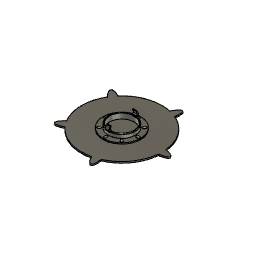
Spool Painting Turntable v16 (Autodesk Fusion 360 design; units mm, degrees)
Autodesk Fusion 360 part; units mm, degrees
sketch "Skizze1" plane through (0, 0, 0) normal (0, 0, 1) x (1, 0, 0)
  circle A0 centre (0, 0) radius 25
  circle A1 centre (0, 0) radius 35
  circle A2 centre (0, 0) radius 75
  dimension "d1" = 50
  dimension "d2" = 10
  dimension "d62" = 150
  constraint coincident A0.centre A1.centre
  measures "d1" diameter of A0
  measures "d62" diameter of A2
ref_plane "Arbeitsebene1" through (0, 0, 38) normal (0, 0, 1) x (1, 0, 0)
extrude "Extrusion1" add sketch "Skizze1" against normal blind 2.5 contours A0 | A1 makes body 1
extrude "Extrusion2" add sketch "Skizze1" along normal blind 2 contours A1 bodies 1
extrude "Extrusion3" add sketch "Skizze1" along normal blind 10 contours A0 bodies 1
ref_plane "Arbeitsebene2" through (0, 0, -0.25) normal (0, 0, 1) x (1, 0, 0)
ref_plane "Arbeitsebene3" through (0, 0, 0.75) normal (0, 0, 1) x (1, 0, 0)
sketch "Skizze3" plane through (0, 0, 0.75) normal (0, 0, 1) x (1, 0, 0)
  line L0 (26.5008, 0) -> (33.4992, 0)
  ellipse E0 centre (30, -0.0006) end of major axis (33.4992, 0.0943) minor radius 2.4634 (26.5008, 0) -> (33.4992, 0) ccw
  spline S0 degree 3 poles (26.2062, 0) (26.2011, -0.4095) (26.3084, -0.8192) (26.5335, -1.1819) (27.1314, -2.1455) (28.4885, -2.7525) (29.8861, -2.7647) (31.1287, -2.7755) (32.3771, -2.3228) (33.1103, -1.5544) (33.5338, -1.1106) (33.7749, -0.5554) (33.795, 0) knots 3.105722 3.105722 3.105722 3.105722 3.531227 3.531227 3.531227 4.661503 4.661503 4.661503 5.666491 5.666491 5.666491 6.246998 6.246998 6.246998 6.246998
  line L1 (26.2062, 0) -> (33.795, 0)
revolve "Drehen5" add sketch "Skizze3" angle 360 about axis through (26.5008, 0, 0.75) along (1, 0, 0) separate body contours L0 E0 L1 makes body 2
revolve "Drehen6" add sketch "Skizze3" angle 360 about axis through (26.2062, 0, 0.75) along (1, 0, 0) separate body makes body 3
pattern_circular "C-Anordnung1" count 8 over 360 about axis through (0, 0, 1.75) along (0, 0, 1) of bodies 3 2 makes body 4 at (22.2285, 20.1064, -1.2055) makes body 5 at (0.3217, 29.9358, 3.1938) makes body 6 at (-21.6185, 20.7163, -1.6309) makes body 7 at (-29.9358, -0.638, 3.1309) makes body 8 at (-19.4839, -22.851, 1.388) makes body 9 at (-0.3217, -29.9358, 3.1938) makes body 10 at (20.1064, -22.2285, -1.2055) makes body 11 at (22.6983, 19.5962, -0.9331) makes body 12 at (2.1935, 29.9035, -0.9331) makes body 13 at (-19.5962, 22.6983, -0.9331) makes body 14 at (-29.9035, -0.7156, -1.9206) makes body 15 at (-19.9571, -22.3374, -1.4435) makes body 16 at (-2.1935, -29.9035, -0.9331) makes body 17 at (19.5962, -22.6983, -0.9331)
combine "Kombinieren3" operation cut target body 1 tool bodies 3 14 17 16 15 12 13 11
fillet "Abrundung1" radius 1.75 1 edges at (-23.3082, -9.0404, 10) on bodies 1
sketch "Skizze5" plane through (0, 0, 10) normal (0, 0, 1) x (-1, 0, 0)
  circle A0 centre (0, 0) radius 23.25
  circle A1 centre (0, 0) radius 23
  dimension "d34" = 46
  constraint coincident A0.centre A1.centre
  measures "d34" diameter of A1
extrude "Extrusion6" cut sketch "Skizze5" against normal up to surface (10.5 mm away) contours A1 bodies 1
fillet "Abrundung4" radius 0.75 1 edges at (21.4435, -8.3172, 10) on bodies 1
ref_plane "Arbeitsebene4" through (0, 0, -1.7) normal (0, 0, -1) x (-1, 0, 0)
sketch "Skizze6" plane through (0, 0, -1.7) normal (0, 0, -1) x (1, 0, 0)
  line L0 (-34, 0.2) -> (-26, 0.2)
  line L1 (-26, 0.2) -> (-26, -0.2)
  line L2 (-26, -0.2) -> (-34, -0.2)
  line L3 (-34, -0.2) -> (-34, 0.2)
  line L4 (-30.2, 3) -> (-29.8, 3)
  line L5 (-29.8, 3) -> (-29.8, -3)
  line L6 (-29.8, -3) -> (-30.2, -3)
  line L7 (-30.2, -3) -> (-30.2, 3)
  constraint horizontal L0
  constraint vertical L1
  constraint horizontal L2
  constraint vertical L3
  constraint horizontal L4
  constraint vertical L5
  constraint horizontal L6
  constraint vertical L7
extrude "Extrusion8" add sketch "Skizze6" against normal blind 0.2 separate body makes body 18
pattern_circular "C-Anordnung3" count 8 over 360 about axis through (0, 0, 1.75) along (0, 0, 1) of bodies 18 makes body 19 at (-19.2333, -19.3276, -1.7) makes body 20 at (0.0667, -32.7333, -1.7) makes body 21 at (19.3276, -19.2333, -1.7) makes body 22 at (31.4667, -0.0667, -1.7) makes body 23 at (19.2333, 19.3276, -1.7) makes body 24 at (-0.0667, 32.7333, -1.7) makes body 25 at (-19.3276, 19.2333, -1.7)
sketch "Skizze7" plane through (0, 0, 0) normal (1, 0, 0) x (0, 1, 0)
  line L0 (25, 8) -> (25, 9.8126)
  line L1 (25.1778, 10.0593) -> (27.8222, 10.9407)
  line L2 (28, 11.1874) -> (28, 11.9386)
  line L3 (27.9726, 12.0549) -> (25.0719, 17.8563)
  line L4 (24.8393, 18) -> (23.4207, 18)
  line L5 (23.1881, 17.6237) -> (25.8659, 12.2681)
  line L6 (25.7156, 11.9052) -> (23.1778, 11.0593)
  line L7 (23, 10.8126) -> (23, 8)
  line L8 (23, 8) -> (25, 8)
  arc A0 (27.8222, 10.9407) -> (28, 11.1874) centre (27.74, 11.1874) ccw
  arc A1 (28, 11.9386) -> (27.9726, 12.0549) centre (27.74, 11.9386) ccw
  arc A2 (25.0719, 17.8563) -> (24.8393, 18) centre (24.8393, 17.74) ccw
  arc A3 (23.4207, 18) -> (23.1881, 17.6237) centre (23.4207, 17.74) ccw
  arc A4 (25.7156, 11.9052) -> (25.8659, 12.2681) centre (25.6334, 12.1519) ccw
  arc A5 (23.1778, 11.0593) -> (23, 10.8126) centre (23.26, 10.8126) ccw
  arc A6 (25.1778, 10.0593) -> (25, 9.8126) centre (25.26, 9.8126) ccw
  dimension "d57" = 0.26
  constraint vertical L0
  constraint parallel L0 L2
  constraint perpendicular L2 L4
  constraint parallel L3 L5
  constraint vertical L7
  constraint perpendicular L0 L8
  constraint tangent L1 A0
  constraint tangent L2 A0
  constraint tangent L2 A1
  constraint tangent L3 A1
  constraint equal A0 A1
  constraint tangent L3 A2
  constraint tangent L4 A2
  constraint equal A0 A2
  constraint tangent L4 A3
  constraint tangent L5 A3
  constraint equal A0 A3
  constraint tangent L5 A4
  constraint tangent L6 A4
  constraint equal A0 A4
  constraint tangent L6 A5
  constraint tangent L7 A5
  constraint equal A0 A5
  constraint tangent L0 A6
  constraint tangent L1 A6
  constraint equal A0 A6
  measures "d57" radius of A0
extrude "Extrusion9" add sketch "Skizze7" along normal mid plane 7 separate body makes body 26
pattern_circular "C-Anordnung4" count 2 over 360 about axis through (0, 0, 1.75) along (0, 0, 1) of bodies 26 makes body 27
extrude "Extrusion10" add sketch "Skizze1" against normal up to surface (2.5 mm away) contours A2 bodies 1
sketch "Skizze8" plane through (0, 0, 0) normal (0, 0, 1) x (-1, 0, 0)
  circle A0 centre (0, 0) radius 35
  circle A1 centre (0, 0) radius 75
  spline S0 degree 2 poles (-74.6288, -7.4526) (-120, 0) (-74.7004, 6.6971) knots 0 0 0 3.405699 3.405699 3.405699 weights 1 0.518951 1
  constraint coincident A1 S0.end
  constraint coincident A1 S0.start
extrude "Extrusion11" add sketch "Skizze8" against normal up to surface (2.5 mm away) separate body contours A1 S0 makes body 28
pattern_circular "C-Anordnung5" count 5 over 360 about axis through (0, 0, 1.75) along (0, 0, 1) of bodies 28 makes body 29 at (24.7604, 75.6504, 0) makes body 30 at (-63.9452, 46.8331, 0) makes body 31 at (-64.301, -46.3431, 0) makes body 32 at (24.4367, -75.7586, 0)
combine "Kombinieren4" operation add target body 1 tool bodies 31 30 32 28 29
equation "d62 = ( 75 * 2 ) * 1 mm"
named bodies: "Base", "Rolle", "Rolle Spiel", "Rolle (1)", "Rolle (2)", "Rolle (3)", "Rolle (4)", "Rolle (5)", "Rolle (6)", "Rolle (7)", "Rolle Spiel (1)", "Rolle Spiel (2)", "Rolle Spiel (3)", "Rolle Spiel (4)", "Rolle Spiel (5)", "Rolle Spiel (6)", "Rolle Spiel (7)", "Support", "Support (1)", "Support (2)", "Support (3)", "Support (4)", "Support (5)", "Support (6)", "Support (7)", "Fixierung", "Fixierung (1)", "Eselsohr", "Eselsohr (1)", "Eselsohr (2)", "Eselsohr (3)", "Eselsohr (4)"
